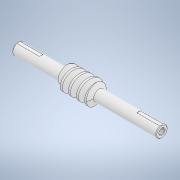
# Autodesk Inventor part: Worm
Saved by Autodesk Inventor 2020 (Build 240168000, 168)
## iProperties
CustomPartVersion: 0
Created: 2020-05-17
Part Number: Worm
Material: Acetal Resin, White
Document SubType Name: Modeling
Designer: Hesekiel
Categories: <?xml version="1.0" encoding="UTF-16"?> <MemberInstance><Categories><FamilyTemplate><FamilyTemplateParameter ValueType="xs:double" Id="1" ObjectReferenceKey="da_z" ObjectType="kUserParameterObject"/><FamilyTemplateParameter ValueType="xs:double" Id="2" ObjectReferenceKey="da_b" ObjectType="kUserParameterObject"/><FamilyTemplateParameter ValueType="xs:double" Id="3" ObjectReferenceKey="da_beta" ObjectType="kUserParameterObject"/><FamilyTemplateParameter ValueType="xs:double" Id="4" ObjectReferenceKey="da_m" ObjectType="kUserParameterObject"/><FamilyTemplateParameter ValueType="xs:double" Id="5" ObjectReferenceKey="da_alpha" ObjectType="kUserParameterObject"/><FamilyTemplateParameter ValueType="xs:double" Id="6" ObjectReferenceKey="da_da" ObjectType="kUserParameterObject"/><FamilyTemplateParameter ValueType="xs:double" Id="7" ObjectReferenceKey="da_aw" ObjectType="kUserParameterObject"/><FamilyTemplateParameter ValueType="xs:double" Id="8" ObjectReferenceKey="da_px" ObjectType="kUserParameterObject"/><FamilyTemplateParameter ValueType="xs:double" Id="9" ObjectReferenceKey="da_d" ObjectType="kUserParameterObject"/><FamilyTemplateParameter ValueType="xs:string" Id="10" ObjectReferenceKey="EAIAABAAAADKGAAAAAAAAIAAAAAAAAAA" ObjectType="83910656" SubObjectId="SurfaceGeometry"/></FamilyTemplate><ParamToTemplateMap><ParamToTemplate CategoryParameter="//CategoryParameter[@InternalName='046C89C9-8512-4d59-83FE-43B91F4F132A']" TemplateParameter="1"/><ParamToTemplate CategoryParameter="//CategoryParameter[@InternalName='2552DF32-E462-4b46-AEBF-C6C7768E72AC']" TemplateParameter="2"/><ParamToTemplate CategoryParameter="//CategoryParameter[@InternalName='C9EE641D-15FC-4fae-A226-E94C4372FDD7']" TemplateParameter="3"/><ParamToTemplate><ParamToTemplate CategoryParameter="//CategoryParameter[@InternalName='00B6519A-459B-49c7-AD84-2E56D39A5744']" ConstantValue="0.000000"/></ParamToTemplate><ParamToTemplate><ParamToTemplate CategoryParameter="//CategoryParameter[@InternalName='04B31F0E-C7A6-4894-AA32-9629BEFACF47']" ConstantValue="1.000000"/></ParamToTemplate><ParamToTemplate><ParamToTemplate CategoryParameter="//CategoryParameter[@InternalName='43CBEC2E-7847-49e7-A936-2F7889FCB2D9']" ConstantValue="0.200000"/></ParamToTemplate><ParamToTemplate><ParamToTemplate CategoryParameter="//CategoryParameter[@InternalName='B1EFC894-105D-4ebd-86BF-FA20ED196853']" ConstantValue="0.300000"/></ParamToTemplate><ParamToTemplate><ParamToTemplate CategoryParameter="//CategoryParameter[@InternalName='51175063-3D10-4879-93E8-6246FE8B403D']" ConstantValue="2067000000.000000"/></ParamToTemplate><ParamToTemplate><ParamToTemplate CategoryParameter="//CategoryParameter[@InternalName='A3A52E27-4454-46a9-B0BD-C932399B70AF']" ConstantValue="0.270000"/></ParamToTemplate><ParamToTemplate CategoryParameter="//CategoryParameter[@InternalName='91B76062-C214-41d9-B1B9-14D2AB99603D']" TemplateParameter="4"/><ParamToTemplate CategoryParameter="//CategoryParameter[@InternalName='2D373A89-B862-43d6-8D0B-0CBF12AB9F6C']" TemplateParameter="5"/><ParamToTemplate CategoryParameter="//CategoryParameter[@InternalName='37777632-D6A2-4fac-9D53-DB8ACD95C989']" TemplateParameter="6"/><ParamToTemplate CategoryParameter="//CategoryParameter[@InternalName='FD1017F1-B727-4f7e-9707-0F86F1FF9423']" TemplateParameter="7"/><ParamToTemplate CategoryParameter="//CategoryParameter[@InternalName='3BF567DA-17EF-48d8-80EA-D119B07F6463']" TemplateParameter="8"/><ParamToTemplate CategoryParameter="//CategoryParameter[@InternalName='BF5A1E7E-5373-4a22-AAD3-F583781FCF3C']" TemplateParameter="9"/><ParamToTemplate><ParamToTemplate CategoryParameter="//CategoryParameter[@InternalName='D4F72237-D604-435a-AD0B-F738B7463A00']" ConstantValue="1.000000"/></ParamToTemplate><ParamToTemplate CategoryParameter="//CategoryParameter[@InternalName='27C3BAF2-7550-4e4b-AE2C-0DB134B7D9B7']" TemplateParameter="10"/></ParamToTemplateMap><Category DisplayName="Gear" InternalName="DC85795E-93AB-48d5-8EEE-5A27447B64BD" Mnemonic="Gear"><CategoryParameter DisplayName="z" InternalName="046C89C9-8512-4d59-83FE-43B91F4F132A" Mnemonic="z"/><CategoryParameter DisplayName="b|.1|" InternalName="2552DF32-E462-4b46-AEBF-C6C7768E72AC" Mnemonic="b"/><CategoryParameter DisplayName="||g|" InternalName="C9EE641D-15FC-4fae-A226-E94C4372FDD7" Mnemonic="beta"/><CategoryParameter DisplayName="x" InternalName="00B6519A-459B-49c7-AD84-2E56D39A5744" Mnemonic="x"/><CategoryParameter DisplayName="a*" InternalName="04B31F0E-C7A6-4894-AA32-9629BEFACF47" Mnemonic="a"/><CategoryParameter DisplayName="c*" InternalName="43CBEC2E-7847-49e7-A936-2F7889FCB2D9" Mnemonic="c"/><CategoryParameter DisplayName="r|.f|*" InternalName="B1EFC894-105D-4ebd-86BF-FA20ED196853" Mnemonic="rf"/><CategoryParameter DisplayName="E" InternalName="51175063-3D10-4879-93E8-6246FE8B403D" Mnemonic="E"/><CategoryParameter DisplayName="||m|" InternalName="A3A52E27-4454-46a9-B0BD-C932399B70AF" Mnemonic="mi"/><Category DisplayName="WormGear" InternalName="1B25C7EF-093B-4025-B3D3-619CD2A4550C" Mnemonic="WormGear"><CategoryParameter DisplayName="m" InternalName="91B76062-C214-41d9-B1B9-14D2AB99603D" Mnemonic="m"/><CategoryParameter DisplayName="||a|" InternalName="2D373A89-B862-43d6-8D0B-0CBF12AB9F6C" Mnemonic="alpha"/><CategoryParameter DisplayName="d|.a|" InternalName="37777632-D6A2-4fac-9D53-DB8ACD95C989" Mnemonic="da"/><CategoryParameter DisplayName="a|.w|" InternalName="FD1017F1-B727-4f7e-9707-0F86F1FF9423" Mnemonic="aw"/><CategoryParameter DisplayName="p|.x|" InternalName="3BF567DA-17EF-48d8-80EA-D119B07F6463" Mnemonic="px"/><CategoryParameter DisplayName="d" InternalName="BF5A1E7E-5373-4a22-AAD3-F583781FCF3C" Mnemonic="d"/><CategoryParameter DisplayName="k|.mat|" InternalName="D4F72237-D604-435a-AD0B-F738B7463A00" Mnemonic="Coef"/><CategoryParameter DisplayName="PitchDiameter" InternalName="27C3BAF2-7550-4e4b-AE2C-0DB134B7D9B7" Mnemonic="IDS_PITCHDIAM"/></Category></Category></Categories></MemberInstance>
Density: 1.425 g/cm^3
Appearance: Smooth - White
Mass: 136.603 g
Surface Area: 244.377 cm^2
Volume: 95.8616 cm^3
Author: Hesekiel
Autodesk Inventor part; units mm, degrees
ref_plane "YZ Plane" through (0, 0, 0) normal (1, 0, 0) x (0, 1, 0)
ref_plane "XY Plane" through (0, 0, 0) normal (0, 0, 1) x (1, 0, 0)
sketch "Base Body Sketch" plane through (0, 0, 0) normal (1, 0, 0) x (0, 1, 0)
  circle A0 centre (0, 0) radius 18.675
  dimension "d5" = 37.35
extrude "Base Body" add sketch "Base Body Sketch" along normal mid plane 60
sketch "Sketch5" plane through (30, 0, 0) normal (1, 0, 0) x (0, 0, -1)
  circle A0 centre (0, 0) radius 18.675 projected
  circle A1 centre (0, 0) radius 14.175
  dimension "d59" = 28.35
  constraints: 1 centre point, 1 coincident
  measures "d59" diameter of A1
surface extrude "Pitch Diameter" sketch "Sketch5" against normal through all shown no curves A1
chamfer "Chamfer1" distance 3.6033 distance2 9.9 1 edges at (30, -18.675, 0) measured on face at (29.5, -18.675, 0)
chamfer "Chamfer2" distance 3.6033 distance2 9.9 1 edges at (-30, -18.675, 0) measured on face at (-29.5, -18.675, 0)
sketch "Tooth Sketch" plane through (0, 0, 0) normal (0, 0, 1) x (1, 0, 0)
  line L0 (0, 22.6341) -> (0, -3.7724) projected
  line L1 (-54.7202, 18.8618) -> (-51.0489, 8.775)
  line L2 (-47.9112, 8.775) -> (-44.24, 18.8618)
  line L3 (-87.6643, 0) -> (142.944, 0) projected
  line L4 (-54.7202, 18.8618) -> (-49.4801, 18.8618)
  line L5 (-49.4801, 18.8618) -> (-44.24, 18.8618)
  line L6 (-51.0489, 8.775) -> (-49.4801, 8.775)
  line L7 (-49.4801, 8.775) -> (-47.9112, 8.775)
  line L8 (-49.4801, 14.175) -> (-45.9458, 14.175) construction
  line L9 (-49.4801, 18.8618) -> (-49.4801, 8.775) construction
  dimension "d24" = 110
  dimension "d25" = 49.4801
  dimension "d26" = 3.5343
  dimension "d27" = 8.775
  dimension "d28" = 14.175
  dimension "d29" = 18.8618
  constraints: 16 end point, 3 equal length, 3 parallel, 2 collinear, 2 point on line
  measures "d24" angle of L6 L1
  measures "d25" distance from line of L0 L4.end
  measures "d26" distance of L8.start L8.end
  measures "d27" distance between parallel lines of L3 L6
  measures "d28" distance between parallel lines of L3 L8
  measures "d29" distance between parallel lines of L3 L4
feature "Tooth" [suppressed]
pattern_circular "Tooth Pattern" [suppressed]
coil "Left Tooth" sketch "Tooth Sketch" operation cut axis through (-10, 0, 0) along (1, 0, 0) pitch 14.1372 turns 7 hand left
pattern_of_one "Left Tooth Pattern"
sketch "Sketch6" plane through (30, 0, 0) normal (1, 0, 0) x (0, 0, -1)
  arc A0 (-0.6111, -8.7537) -> (-8.7252, -0.9333) centre (0, 0) ccw projected
  arc A1 (-8.7252, -0.9333) -> (-0.6111, -8.7537) centre (0, 0) ccw projected
  arc A2 (0.1559, 18.6743) -> (0, 18.675) centre (0, 0) ccw projected
  circle A3 centre (0, 0) radius 10
  point P0 (-18.5691, -1.9864)
  dimension "d83" = 20
  constraints: 1 centre point, 1 coincident
  measures "d83" diameter of A3
extrude "Extrusion2" add sketch "Sketch6" along normal blind 50 contours A1 A0 | A3
sketch "Sketch7" plane through (80, 0, 0) normal (1, 0, 0) x (0, 0, -1)
  circle A0 centre (0, 0) radius 10
  dimension "d84" = 20
  constraints: 1 centre point, 1 coincident
  measures "d84" diameter of A0
extrude "Extrusion3" add sketch "Sketch7" along normal blind 60
sketch "Sketch8" plane through (140, 0, 0) normal (1, 0, 0) x (0, 0, -1)
  circle A0 centre (0, 0) radius 5
  dimension "d87" = 10
  constraints: 1 centre point, 1 coincident
  measures "d87" diameter of A0
extrude "Extrusion4" cut sketch "Sketch8" against normal blind 30
thread "Thread1" size "M10x1.5" class "6H" standard "ANSI Metric M Profile" full length
sketch "Sketch9" plane through (-30, 0, 0) normal (-1, 0, 0) x (0, 0, 1)
  circle A0 centre (0, 0) radius 10
  dimension "d92" = 20
  constraints: 1 centre point, 1 coincident
  measures "d92" diameter of A0
extrude "Extrusion5" add sketch "Sketch9" along normal blind 82.5
chamfer "Chamfer4" distance 0.7 angle 45 1 edges at (140, 0, 5)
sketch "Sketch10" plane through (110, 0, 0) normal (1, 0, 0) x (0, 0, -1)
  point P0 (0, 0)
sketch "Sketch11" plane through (110, 0, 0) normal (1, 0, 0) x (0, 0, -1)
  point P0 (0, 0)
sketch "Sketch12" plane through (110, 0, 0) normal (1, 0, 0) x (0, 0, -1)
  point P0 (0, 0)
sketch "Sketch13" plane through (110, 0, 0) normal (1, 0, 0) x (0, 0, -1)
  point P0 (0, 0)
sketch "Sketch14" plane through (110, 0, 0) normal (1, 0, 0) x (0, 0, -1)
  point P0 (0, 0)
hole "Hole5" at (110, 0, 0) direction (-1, 0, 0) diameter 8.376 depth 5 tip angle 120 thread size "M10x1.5" class "6H" standard "ISO Metric profile"
ref_plane "Work Plane10" through (-30, 10, 0) normal (0, 1, 0) x (-1, 0, 0)
chamfer "Chamfer3" distance 1 angle 45 2 edges at (-112.5, 0, -10) (140, 0, 10)
sketch "Sketch15" plane through (-30, 10, 0) normal (0, 1, 0) x (-1, 0, 0)
  line L0 (0, -10) -> (0, 10) projected
  line L1 (81.5, -10) -> (81.5, 10) projected
  line L2 (-60, 10) -> (-60, -10) projected
  line L3 (-169, 10) -> (-169, -10) projected
  line L4 (81.5, -10) -> (81.5, 10) projected
  line L5 (81.5, 0) -> (81.5, -3)
  line L6 (-169, 10) -> (-169, -10) projected
  line L7 (81.5, -3) -> (-169, -3)
  line L8 (-169, -3) -> (-169, 3)
  line L9 (-169, 3) -> (81.5, 3)
  line L10 (81.5, 3) -> (81.5, -3)
  line L11 (81.5, -3) -> (41.5, -3)
  line L12 (41.5, -3) -> (41.5, 3)
  line L13 (41.5, 3) -> (81.5, 3)
  line L14 (81.5, 3) -> (81.5, -3)
  line L15 (-169, -3) -> (-129, -3)
  line L16 (-129, -3) -> (-129, 3)
  line L17 (-129, 3) -> (-169, 3)
  line L18 (-169, 3) -> (-169, -3)
  point P0 (-30, 0)
  point P1 (81.5, 3)
  dimension "d136" = 3
  dimension "d137" = 6
  dimension "d138" = 40
  dimension "d139" = 40
  dimension "d140" = 6
  constraints: 26 end point, 6 parallel, 3 horizontal, 3 perpendicular, 3 point on line, 1 midpoint
  measures "d136" distance of L5.start L5.end
  measures "d137" distance of L7.end L8.end
  measures "d138" distance of L12.end L13.end
  measures "d139" distance of L17.end L16.end
  measures "d140" distance of L16.end L15.end
extrude "Extrusion6" cut sketch "Sketch15" against normal blind 0.5 contours L12 L9 L1 L7 | L7 L3 L9 L16
sketch "Sketch16" plane through (-111.5, 0, 0) normal (1, 0, 0) x (0, 0, -1)
  arc A0 (3, 9.5394) -> (-3, 9.5394) centre (0, 0) ccw projected
  line L0 (-3, 9.5394) -> (-3, 9.5) projected
  line L1 (-3, 9.5) -> (3, 9.5) projected
  line L2 (3, 9.5394) -> (3, 9.5) projected
extrude "Extrusion7" cut sketch "Sketch16" against normal blind 0.5
sketch "Sketch17" plane through (139, 0, 0) normal (-1, 0, 0) x (0, 0, 1)
  arc A0 (3, 9.5394) -> (-3, 9.5394) centre (0, 0) ccw projected
  line L0 (-3, 9.5394) -> (-3, 9.5) projected
  line L1 (-3, 9.5) -> (3, 9.5) projected
  line L2 (3, 9.5394) -> (3, 9.5) projected
extrude "Extrusion8" cut sketch "Sketch17" against normal blind 0.5
equation "\"d6\" = da_b"
equation "\"d8\" = fd_cham1"
equation "\"d9\" = 0.5 * fd_cham2"
equation "\"d10\" = fd_cham1"
equation "\"d11\" = 0.5 * fd_cham2"
equation "\"d25\" = fd_dist"
equation "\"d26\" = 0.25 * da_px"
equation "\"d27\" = 0.5 * da_df"
equation "\"d28\" = 0.5 * da_d"
equation "\"d29\" = 0.505 * da_da"
equation "\"d32\" = fd_n"
equation "\"da_rightdir\" = 0"
equation "\"d64\" = fd_n"
equation "\"d5\" = da_da"
equation "\"d59\" = da_d"
equation "\"da_b\" = 60"
equation "\"da_df\" = 17.55"
equation "\"da_da\" = 37.35"
equation "\"fd_cham2\" = da_da - da_df"
equation "\"fd_cham1\" = 0.181985 * fd_cham2"
equation "\"da_d\" = 28.35"
equation "\"da_px\" = 14.137167"
equation "\"da_alfat\" = 20deg"
equation "\"fd_dist\" = 49.480084"
equation "\"fd_n\" = 7"
body "Solid1"
body "Srf1"
